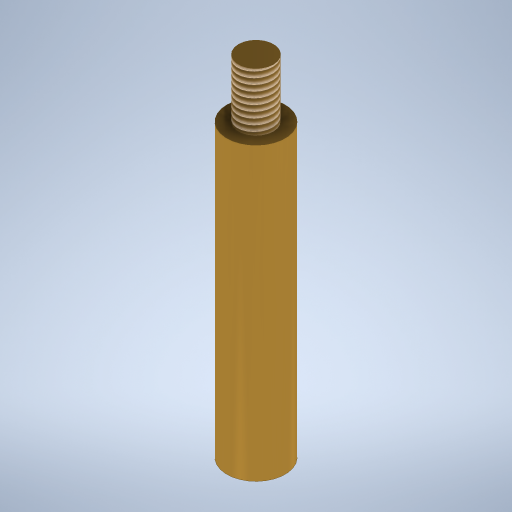
# Autodesk Inventor part: Fitting-3
Saved by Autodesk Inventor 2024 (Build 280153000, 153)
## iProperties
Created: 2023-09-24
Part Number: Fitting-3
Material: Brass
Document SubType Name: Modeling
Designer: schanen
Density: 8.49 g/cm^3
Appearance: Brass - Polished
Author: schanen
Autodesk Inventor part; units mm, degrees
ref_plane "YZ Plane" through (0, 0, 0) normal (1, 0, 0) x (0, 1, 0)
ref_plane "XZ Plane" through (0, 0, 0) normal (0, 1, 0) x (-1, 0, 0)
ref_plane "XY Plane" through (0, 0, 0) normal (0, 0, 1) x (1, 0, 0)
sketch "Sketch1" plane through (0, 0, 0) normal (0, 0, 1) x (1, 0, 0)
  line L0 (0, 24) -> (-1.5, 24)
  line L1 (-1.5, 24) -> (-1.5, 19)
  line L2 (-1.5, 19) -> (-2.5, 19)
  line L3 (-2.5, 19) -> (-2.5, -6)
  line L4 (-2.5, -6) -> (-1.5, -6)
  line L5 (-1.5, -6) -> (-1.5, 0)
  line L6 (-1.5, 0) -> (0, 0)
  line L7 (0, 0) -> (0, 24)
  dimension "d0" = 1.5
  dimension "d2" = 2.5
  dimension "d4" = 5
  dimension "d5" = 25
  dimension "d9" = 6
  constraints: 16 end point, 6 perpendicular, 2 vertical alignment, 1 coincident, 1 horizontal, 1 vertical
  measures "d0" distance between parallel lines of L7 L1
  measures "d2" distance between parallel lines of L7 L3
  measures "d4" distance of L0.end L1.end
  measures "d5" distance of L2.end L3.end
  measures "d9" distance of L4.end L5.end
revolve "Revolution1" add sketch "Sketch1" angle 360 about axis through (0, 0, 0) along (0, 1, 0)
thread "Thread1" size "M3x0.5" class "6g" standard "ANSI Metric M Profile" full length
thread "Thread2" size "M3x0.5" class "6H" standard "ANSI Metric M Profile" full length
body "Solid1"
